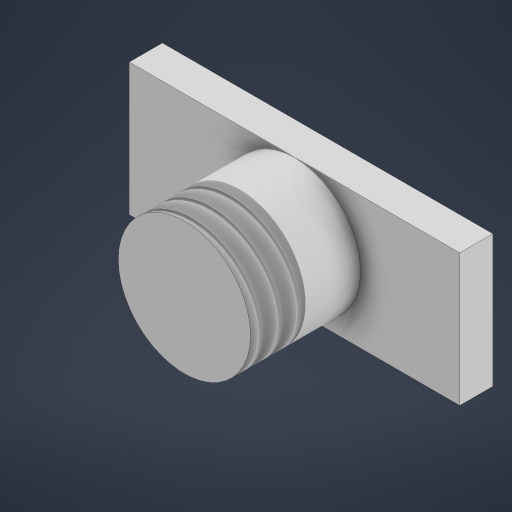
# Autodesk Inventor part: BOTTOM STOPPER
Saved by Autodesk Inventor 2023 (Build 270158000, 158)
## iProperties
Created: 2023-12-28
Part Number: BOTTOM STOPPER
Material: Generic
Document SubType Name: Modeling
Designer: User
Density: 1 g/cm^3
Appearance: Default
Author: User
Autodesk Inventor part; units mm, degrees
ref_plane "YZ Plane" through (0, 0, 0) normal (1, 0, 0) x (0, 1, 0)
ref_plane "XZ Plane" through (0, 0, 0) normal (0, 1, 0) x (-1, 0, 0)
ref_plane "XY Plane" through (0, 0, 0) normal (0, 0, 1) x (1, 0, 0)
sketch "Sketch1" plane through (0, 0, 0) normal (0, 0, 1) x (1, 0, 0)
  line L0 (-15, 6) -> (15, 6)
  line L1 (15, 6) -> (15, -6)
  line L2 (15, -6) -> (-15, -6)
  line L3 (-15, -6) -> (-15, 6)
  line L4 (-15, 6) -> (15, -6) construction
  line L5 (15, 6) -> (-15, -6) construction
  point P0 (0, 0)
  dimension "d0" = 30
  dimension "d1" = 12
  constraints: 12 end point, 2 midpoint, 2 parallel, 1 horizontal, 1 perpendicular
  measures "d0" distance of L1.end L2.end
  measures "d1" distance of L0.end L1.end
extrude "Extrusion1" add sketch "Sketch1" along normal blind 3
sketch "Sketch2" plane through (0, 0, 3) normal (0, 0, 1) x (1, 0, 0)
  circle A0 centre (0, 0) radius 6
  dimension "d4" = 12
  constraints: 1 centre point, 1 coincident
  measures "d4" diameter of A0
extrude "Extrusion2" add sketch "Sketch2" along normal blind 10
thread "Thread2" size "M12x1.75" class "6g" standard "ANSI Metric M Profile" length 5
body "Solid1"
